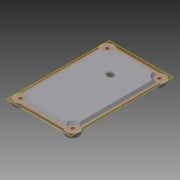
# Autodesk Inventor part: Projectenclosurelid
Saved by Autodesk Inventor 2015 (Build 190159000, 159)
## iProperties
Created: 2015-06-17
Part Number: Projectenclosurelid
Material: Generic
Document SubType Name: Modeling
Designer: Hunter
Density: 1 g/cm^3
Appearance: Default
Author: Hunter
Autodesk Inventor part; units mm, degrees
ref_plane "YZ Plane" through (0, 0, 0) normal (1, 0, 0) x (0, 1, 0)
ref_plane "XZ Plane" through (0, 0, 0) normal (0, 1, 0) x (-1, 0, 0)
ref_plane "XY Plane" through (0, 0, 0) normal (0, 0, 1) x (1, 0, 0)
sketch "Sketch1" plane through (0, 0, 0) normal (0, 1, 0) x (-1, 0, 0)
  line L0 (0, 0) -> (82.55, 0)
  line L1 (82.55, 0) -> (82.55, 133.35)
  line L2 (82.55, 133.35) -> (0, 133.35)
  line L3 (0, 133.35) -> (0, 0)
  dimension "d0" = 133.35
  dimension "d1" = 82.55
  constraints: 8 end point, 2 parallel, 1 horizontal, 1 perpendicular
  measures "d0" distance of L0.end L1.end
  measures "d1" distance of L1.end L2.end
extrude "Extrusion1" add sketch "Sketch1" along normal blind 6.35
sketch "Sketch3" plane through (0, 0, 0) normal (0, -1, 0) x (1, 0, 0)
  circle A0 centre (-3.175, 130.175) radius 6.35
  circle A1 centre (-3.175, 3.175) radius 6.35
  circle A2 centre (-79.375, 3.175) radius 6.35
  circle A3 centre (-79.375, 130.175) radius 6.35
  point P0 (0, 0)
  dimension "d14" = 12.7
  dimension "d15" = 12.7
  dimension "d16" = 12.7
  dimension "d17" = 12.7
  constraints: 4 centre point
  measures "d14" diameter of A0
  measures "d15" diameter of A1
  measures "d16" diameter of A2
  measures "d17" diameter of A3
extrude "Extrusion2" cut sketch "Sketch3" against normal blind 6.35
chamfer "Chamfer3" distance 3.175 angle 45 8 edges at (-74.8849, 6.35, 125.6849) (-7.6651, 6.35, 125.6849) (0, 6.35, 66.675) (-7.6651, 6.35, 7.6651) (-41.275, 6.35, 0) (-74.8849, 6.35, 7.6651) (-82.55, 6.35, 66.675) (-41.275, 6.35, 133.35)
fillet "Fillet2" radius 3.175 2 edges at (-10.6871, 4.5498, 1.3748) (-1.3748, 4.5498, 10.6871)
fillet "Fillet3" radius 3.175 6 edges at (-10.6871, 4.5498, 131.9752) (-1.3748, 4.5498, 122.6629) (-71.8629, 4.5498, 1.3748) (-81.1752, 4.5498, 10.6871) (-71.8629, 4.5498, 131.9752) (-81.1752, 4.5498, 122.6629)
ref_plane "Work Plane1" through (0, 3.175, 100.0125) normal (0, 1, 0) x (0, 0, -1)
sketch "Sketch4" plane through (0, 3.175, 100.0125) normal (0, 1, 0) x (0, 0, -1)
  arc A0 (100.0125, 8.6743) -> (91.3382, 0) centre (96.8375, 3.175) ccw projected
  circle A1 centre (96.8375, 3.175) radius 9.525
  arc A2 (91.3382, 82.55) -> (100.0125, 73.8757) centre (96.8375, 79.375) ccw projected
  circle A3 centre (96.8375, 79.375) radius 9.525
  arc A4 (-23.8498, 2.488) -> (-30.8495, 9.4877) centre (-30.1625, 3.175) ccw projected
  circle A5 centre (-30.1625, 3.175) radius 9.525
  arc A6 (-30.8495, 73.0623) -> (-23.8498, 80.062) centre (-30.1625, 79.375) ccw projected
  circle A7 centre (-30.1625, 79.375) radius 9.525
  point P0 (100.0125, 0)
  dimension "d26" = 19.05
  dimension "d27" = 19.05
  dimension "d28" = 19.05
  dimension "d29" = 19.05
  constraints: 4 centre point, 4 coincident
  measures "d26" diameter of A1
  measures "d27" diameter of A3
  measures "d28" diameter of A7
  measures "d29" diameter of A5
extrude "Extrusion3" add sketch "Sketch4" against normal blind 7.62
fillet "Fillet5" radius 3.175 4 edges at (-3.175, -4.445, 12.7) (-3.175, -4.445, 139.7) (-79.375, -4.445, 139.7) (-79.375, -4.445, 12.7)
sketch "Sketch5" plane through (0, 0, 0) normal (0, -1, 0) x (1, 0, 0)
  arc A0 (0, 121.1947) -> (-12.1553, 133.35) centre (-3.175, 130.175) ccw projected
  circle A1 centre (-79.375, 3.175) radius 9.525 projected
  line L0 (3.1218, 137.3218) -> (-85.7086, 137.3218)
  line L1 (-85.7086, 137.3218) -> (-85.7086, -3.9392)
  line L2 (-85.7086, -3.9392) -> (3.1218, -3.9392)
  line L3 (3.1218, -3.9392) -> (3.1218, 137.3218)
  point P0 (0, 0)
  point P1 (-82.55, 12.1553)
  point P2 (-70.3947, 0)
  constraints: 8 end point, 2 parallel, 2 point on circle, 1 horizontal, 1 perpendicular
extrude "Extrusion4" add sketch "Sketch5" against normal up to surface (3.175 mm away) contours L3 L2 A1 L1 L0 | L2 L1 A1
hole "Hole1" at (-79.375, -4.445, 3.175) direction (0, 1, 0) diameter 5.08 depth 25.4 tip angle 118
hole "Hole3" at (-3.175, -4.445, 3.175) direction (0, 1, 0) diameter 5.08 depth 25.4 tip angle 118
hole "Hole4" at (-3.175, -4.445, 130.175) direction (0, 1, 0) diameter 5.08 depth 25.4 tip angle 118
hole "Hole5" at (-79.375, -4.445, 130.175) direction (0, 1, 0) diameter 5.08 depth 25.4 tip angle 118
fillet "Fillet8" radius 6.35 6 edges at (-70.4644, 0, 126.8095) (-82.7634, 0, 121.2731) (-72.2608, 0, 9.5086) (-10.3055, 0, 9.4902) (-12.0856, 0, 126.8095) (0.1905, 0, 121.2644)
sketch "Sketch6" plane through (0, 6.35, 0) normal (0, 1, 0) x (1, 0, 0)
  circle A0 centre (-41.275, -36.195) radius 3.81
  line L0 (-79.375, -118.621) -> (-79.375, -14.729) projected
  line L1 (-3.175, -14.729) -> (-3.175, -118.621) projected
  line L2 (-67.821, -3.175) -> (-14.729, -3.175) projected
  point P0 (0, 0)
  dimension "d84" = 7.62
  dimension "d87" = 38.1
  dimension "d88" = 33.02
  constraints: 1 centre point
  measures "d84" diameter of A0
  measures "d87" distance from line of L0 A0.centre
  measures "d88" distance from line of L2 A0.centre
extrude "Extrusion5" cut sketch "Sketch6" against normal blind 25.4
fillet "Fillet9" radius 3.175 1 edges at (-45.085, 6.35, 36.195)
sketch "Sketch7" plane through (0, 0, 0) normal (0, -1, 0) x (1, 0, 0)
  point P0 (0, 0)
sketch "Sketch8" plane through (0, 0, 0) normal (0, -1, 0) x (1, 0, 0)
  circle A0 centre (-41.275, 36.195) radius 5.08
  circle A1 centre (-41.275, 36.195) radius 3.81 projected
  point P0 (0, 0)
  dimension "d92" = 10.16
  constraints: 1 centre point, 1 concentric
  measures "d92" diameter of A0
extrude "Extrusion6" add sketch "Sketch8" along normal blind 2.54
fillet "Fillet10" radius 3.175 2 edges at (-46.355, 0, 36.195) (-46.355, -2.54, 36.195)
body "Solid1"
